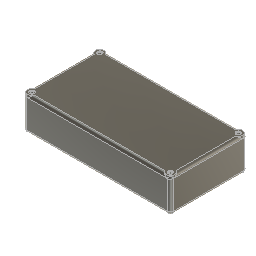
Meadow_Parametric_Enclosure (Autodesk Fusion 360 design; units mm, degrees)
Autodesk Fusion 360 part; units mm, degrees
sketch "Sketch1" plane through (0, 0, 0) normal (0, 0, 1) x (1, 0, 0) in component "Meadow_Enclosure_Bottom"
  line L0 (50, 25) -> (-50, 25)
  line L1 (-50, 25) -> (-50, -25)
  line L2 (-50, -25) -> (50, -25)
  line L3 (50, -25) -> (50, 25)
  line L4 (50, 25) -> (-50, -25) construction
  line L5 (-50, 25) -> (50, -25) construction
  line L6 (-52, -27) -> (52, -27)
  line L7 (52, -27) -> (52, 27)
  line L8 (52, 27) -> (-52, 27)
  line L9 (-52, 27) -> (-52, -27)
  dimension "d5" = 100
  dimension "d6" = 50
  dimension "d7" = 2
  constraint horizontal L0
  constraint perpendicular L0 L1
  constraint parallel L0 L2
  constraint parallel L1 L3
  constraint coincident L4 origin
  constraint coincident L5 origin
  measures "d5" distance of L1.end L2.end
  measures "d6" distance of L0.end L1.end
extrude "Extrude1" add sketch "Sketch1" along normal blind 2 contours L0 L1 L2 L3 makes body 1 in component "Meadow_Enclosure_Bottom"
extrude "Extrude2" add sketch "Sketch1" along normal blind 22 bodies 1 in component "Meadow_Enclosure_Bottom"
fillet "Fillet1" radius 2 8 edges at (-52, -27, 11) (-52, 27, 11) (52, -27, 11) (-52, 0, 0) (0, -27, 0) (0, 27, 0) (52, 0, 0) (52, 27, 11) on bodies 1 in component "Meadow_Enclosure_Bottom"
sketch "Sketch2" plane through (0, 0, 2) normal (0, 0, 1) x (-1, 0, 0) in component "Meadow_Enclosure_Bottom"
  line L0 (-50, 25) -> (-50, -25)
  line L1 (-50, -25) -> (50, -25)
  line L2 (50, -25) -> (50, 25)
  line L3 (50, 25) -> (-50, 25)
  line L4 (42.46, -25) -> (42.46, 25) construction
  line L5 (-50, 12.46) -> (50, 12.46) construction
  point P0 (42.46, 12.46)
  dimension "d148" = 7.54
  dimension "d149" = 12.54
  constraint coincident L1 L4.start
  constraint coincident L3 L4.end
  constraint perpendicular L3 L4
  constraint coincident L0 L5.start
  constraint coincident L2 L5.end
  constraint perpendicular L2 L5
  constraint coincident L4 P0
  constraint coincident L5 P0
  measures "d148" distance of L2.end L4
  measures "d149" distance of L2.end L5
sketch "Sketch6" plane through (0, 0, 22) normal (0, 0, 1) x (-1, 0, 0) in component "Meadow_Enclosure_Bottom"
  line L0 (-50, -25) -> (-50, 25)
  line L1 (-50, 25) -> (50, 25)
  line L2 (50, 25) -> (50, -25)
  line L3 (50, -25) -> (-50, -25)
  arc A0 (52, 25) -> (50, 27) centre (50, 25) ccw
  line L4 (50, 27) -> (-50, 27)
  arc A1 (-50, 27) -> (-52, 25) centre (-50, 25) ccw
  line L5 (-52, 25) -> (-52, -25)
  arc A2 (-52, -25) -> (-50, -27) centre (-50, -25) ccw
  line L6 (-50, -27) -> (50, -27)
  arc A3 (50, -27) -> (52, -25) centre (50, -25) ccw
  line L7 (52, -25) -> (52, 25)
  line L8 (-50, -25) -> (50, -25)
  line L9 (50, -25) -> (50, 25)
  circle A4 centre (49, -24) radius 3
  line L10 (-52, -27) -> (52, -27)
  line L11 (52, -27) -> (52, 27)
  circle A5 centre (49, 24) radius 3
  circle A6 centre (-49, 24) radius 3
  circle A7 centre (-49, -24) radius 3
  line L12 (52, 27) -> (-52, 27)
  line L13 (-52, 27) -> (-52, -27)
  constraint tangent A4 L10
  constraint tangent A4 L11
  constraint tangent L11 A5
  constraint tangent A5 L12
  constraint tangent A6 L13
  constraint tangent A6 L12
  constraint tangent L10 A7
  constraint tangent A7 L13
extrude "Extrude5" add sketch "Sketch6" against normal blind 4 contours L0 L3 L8 A7 | L0 L3 L8 A7 | L0 L1 A6 | L0 L1 A6 | L2 L3 L8 L9 A4 | L2 L3 L8 L9 A4 | L1 L2 L9 A5 | L1 L2 L9 A5 bodies 1 in component "Meadow_Enclosure_Bottom"
fillet "Fillet2" radius 1.5 16 edges at (46.1716, 25, 20) (50, 23.0858, 18) (48.0858, 25, 18) (50, 21.1716, 20) (50, -23.0858, 18) (48.0858, -25, 18) (46.1716, -25, 20) (50, -21.1716, 20) (-46.1716, -25, 20) (-50, -21.1716, 20) (-50, -23.0858, 18) (-48.0858, -25, 18) (-50, 23.0858, 18) (-48.0858, 25, 18) (-46.1716, 25, 20) (-50, 21.1716, 20) on bodies 1 in component "Meadow_Enclosure_Bottom"
hole "Hole2" at (-49, 24, 22) at (49, 24, 22) at (-49, -24, 22) at (49, -24, 22) direction (0, 0, -1) diameter 1.9 depth 3.75 tip angle 180 counterbore diameter 3.4 counterbore depth 3 bodies 1 in component "Meadow_Enclosure_Bottom"
sketch "PCB" plane through (0, 0, 0) normal (0, 0, 1) x (1, 0, 0) in component "Meadow_F7_Micro"
  line L0 (36.83, 11.43) -> (-36.83, 11.43)
  line L1 (-36.83, 11.43) -> (-36.83, -11.43)
  line L2 (-36.83, -11.43) -> (36.83, -11.43)
  line L3 (36.83, -11.43) -> (36.83, 11.43)
  line L4 (36.83, 11.43) -> (-36.83, -11.43) construction
  line L5 (-36.83, 11.43) -> (36.83, -11.43) construction
  circle A0 centre (-34.29, 8.89) radius 1.27
  circle A1 centre (-34.29, -8.89) radius 1.27
  line L6 (-36.83, 0) -> (36.83, 0) construction
  circle A2 centre (34.29, 8.89) radius 1.27
  circle A3 centre (34.29, -8.89) radius 1.27
  line L7 (0, 11.43) -> (0, -11.43) construction
  circle A4 centre (-13.97, 10.16) radius 0.51
  circle A5 centre (-11.43, 10.16) radius 0.51
  circle A6 centre (-8.89, 10.16) radius 0.51
  circle A7 centre (-6.35, 10.16) radius 0.51
  circle A8 centre (-3.81, 10.16) radius 0.51
  circle A9 centre (-1.27, 10.16) radius 0.51
  circle A10 centre (1.27, 10.16) radius 0.51
  circle A11 centre (3.81, 10.16) radius 0.51
  circle A12 centre (6.35, 10.16) radius 0.51
  circle A13 centre (8.89, 10.16) radius 0.51
  circle A14 centre (11.43, 10.16) radius 0.51
  circle A15 centre (13.97, 10.16) radius 0.51
  circle A16 centre (16.51, 10.16) radius 0.51
  circle A17 centre (19.05, 10.16) radius 0.51
  circle A18 centre (-24.13, -10.16) radius 0.51
  circle A19 centre (-21.59, -10.16) radius 0.51
  circle A20 centre (-19.05, -10.16) radius 0.51
  circle A21 centre (-16.51, -10.16) radius 0.51
  circle A22 centre (-13.97, -10.16) radius 0.51
  circle A23 centre (-11.43, -10.16) radius 0.51
  circle A24 centre (-8.89, -10.16) radius 0.51
  circle A25 centre (-6.35, -10.16) radius 0.51
  circle A26 centre (-3.81, -10.16) radius 0.51
  circle A27 centre (-1.27, -10.16) radius 0.51
  circle A28 centre (1.27, -10.16) radius 0.51
  circle A29 centre (3.81, -10.16) radius 0.51
  circle A30 centre (6.35, -10.16) radius 0.51
  circle A31 centre (8.89, -10.16) radius 0.51
  circle A32 centre (11.43, -10.16) radius 0.51
  circle A33 centre (13.97, -10.16) radius 0.51
  circle A34 centre (16.51, -10.16) radius 0.51
  circle A35 centre (19.05, -10.16) radius 0.51
  dimension "d1" = 73.66
  dimension "d2" = 22.86
  dimension "d3" = 2.54
  dimension "d4" = 2.54
  dimension "d5_1" = 2.54
  dimension "d7_1" = 2.54
  dimension "d8" = 1.02
  dimension "d9_1" = 20.32
  dimension "d10_1" = 1.27
  dimension "d13_1" = 2.54
  dimension "d14_1" = 0
  dimension "d15_1" = 1.02
  dimension "d16_1" = 10.16
  dimension "d17_1" = 1.27
  dimension "d20_1" = 2.54
  dimension "d21_1" = 0
  constraint horizontal L0
  constraint perpendicular L0 L1
  constraint parallel L0 L2
  constraint parallel L1 L3
  constraint coincident L4 origin
  constraint coincident L5 origin
  constraint midpoint L1 L6.start
  constraint midpoint L3 L6.end
  constraint symmetric A0.centre A1.centre L6
  constraint equal A0 A2
  constraint equal A0 A3
  constraint midpoint L0 L7.start
  constraint midpoint L2 L7.end
  constraint symmetric A0.centre A2.centre L7
  constraint symmetric A1.centre A3.centre L7
  measures "d1" distance of L1.end L2.end
  measures "d2" distance of L0.end L1.end
  measures "d3" diameter of A0
  measures "d4" distance of L0 A0.centre
  measures "d5_1" distance of L1 A0.centre
  measures "d7_1" diameter of A1
  measures "d8" diameter of A4
  measures "d9_1" horizontal distance of A0.centre A4.centre
  measures "d10_1" distance of L0 A4.centre
  measures "d15_1" diameter of A18
  measures "d16_1" horizontal distance of A1.centre A18.centre
  measures "d17_1" distance of L2 A18.centre
extrude "Extrude1'" add sketch "PCB" against normal blind 1.6 separate body makes body 2 in component "Meadow_F7_Micro"
fillet "Fillet1'" radius 2.54 4 edges at (-36.83, 11.43, -0.8) (-36.83, -11.43, -0.8) (36.83, -11.43, -0.8) (36.83, 11.43, -0.8) on bodies 2 in component "Meadow_F7_Micro"
sketch "Sketch4" plane through (0, 0, 0) normal (0, 0, 1) x (1, 0, 0) in component "Meadow_F7_Micro"
  line L0 (-36.83, 0) -> (36.83, 0) construction
  line L1 (-25.33, 10.93) -> (-18.08, 10.93)
  line L2 (-18.08, 10.93) -> (-18.08, 4.93)
  line L3 (-18.08, 4.93) -> (-25.33, 4.93)
  line L4 (-25.33, 4.93) -> (-25.33, 10.93)
  line L5 (-36.83, 11.43) -> (-36.83, -11.43)
  line L6 (36.83, 11.43) -> (-36.83, 11.43)
  line L7 (9.03, 5) -> (-0.97, 5)
  line L8 (-0.97, 5) -> (-0.97, -5)
  line L9 (-0.97, -5) -> (9.03, -5)
  line L10 (9.03, -5) -> (9.03, 5)
  line L11 (9.03, 5) -> (-0.97, -5) construction
  line L12 (-0.97, 5) -> (9.03, -5) construction
  line L13 (36.83, -11.43) -> (36.83, 11.43)
  line L14 (21.03, 4) -> (15.03, 4)
  line L15 (15.03, 4) -> (15.03, -4)
  line L16 (15.03, -4) -> (21.03, -4)
  line L17 (21.03, -4) -> (21.03, 4)
  line L18 (21.03, 4) -> (15.03, -4) construction
  line L19 (15.03, 4) -> (21.03, -4) construction
  line L20 (29.83, 3.5) -> (22.83, 3.5)
  line L21 (22.83, 3.5) -> (22.83, -3.5)
  line L22 (22.83, -3.5) -> (29.83, -3.5)
  line L23 (29.83, -3.5) -> (29.83, 3.5)
  line L24 (29.83, 3.5) -> (22.83, -3.5) construction
  line L25 (22.83, 3.5) -> (29.83, -3.5) construction
  line L26 (-7.47, -4) -> (-15.47, -4)
  line L27 (-15.47, -4) -> (-15.47, 4)
  line L28 (-15.47, 4) -> (-7.47, 4)
  line L29 (-7.47, 4) -> (-7.47, -4)
  line L30 (-7.47, -4) -> (-15.47, 4) construction
  line L31 (-15.47, -4) -> (-7.47, 4) construction
  line L32 (-22.17, -7.73) -> (-25.67, -7.73)
  line L33 (-25.67, -7.73) -> (-25.67, -1.23)
  line L34 (-25.67, -1.23) -> (-22.17, -1.23)
  line L35 (-22.17, -1.23) -> (-22.17, -7.73)
  line L36 (-22.17, -7.73) -> (-25.67, -1.23) construction
  line L37 (-25.67, -7.73) -> (-22.17, -1.23) construction
  line L38 (-36.83, -11.43) -> (36.83, -11.43)
  line L39 (-32.08, -4) -> (-37.83, -4)
  line L40 (-37.83, -4) -> (-37.83, 4)
  line L41 (-37.83, 4) -> (-32.08, 4)
  line L42 (-32.08, 4) -> (-32.08, -4)
  line L43 (-32.08, -4) -> (-37.83, 4) construction
  line L44 (-37.83, -4) -> (-32.08, 4) construction
  line L45 (34.63, 5.93) -> (36.23, 5.93)
  line L46 (36.23, 5.93) -> (36.23, 2.73)
  line L47 (36.23, 2.73) -> (34.63, 2.73)
  line L48 (34.63, 2.73) -> (34.63, 5.93)
  line L49 (28.23, -7.83) -> (30.83, -7.83)
  line L50 (30.83, -7.83) -> (30.83, -10.43)
  line L51 (30.83, -10.43) -> (28.23, -10.43)
  line L52 (28.23, -10.43) -> (28.23, -7.83)
  line L53 (21.18, 8.13) -> (25.33, 8.13)
  line L54 (25.33, 8.13) -> (25.33, 10.93)
  line L55 (25.33, 10.93) -> (21.18, 10.93)
  line L56 (21.18, 10.93) -> (21.18, 8.13)
  line L57 (21.18, -8.13) -> (25.33, -8.13)
  line L58 (25.33, -8.13) -> (25.33, -10.93)
  line L59 (25.33, -10.93) -> (21.18, -10.93)
  line L60 (21.18, -10.93) -> (21.18, -8.13)
  circle A0 centre (29.53, -9.13) radius 1
  point P0 (4.03, 0)
  point P1 (18.03, 0)
  point P2 (26.33, 0)
  point P3 (-11.47, 0)
  point P4 (-23.92, -4.48)
  point P5 (-34.955, 0)
  dimension "d25" = 7.25
  dimension "d26" = 6
  dimension "d27" = 11.5
  dimension "d28" = 0.5
  dimension "d29" = 10
  dimension "d30" = 10
  dimension "d31" = 27.8
  dimension "d32" = 6
  dimension "d33" = 8
  dimension "d34" = 6
  dimension "d35" = 7
  dimension "d36" = 7
  dimension "d37" = 1.8
  dimension "d38" = 8
  dimension "d39" = 8
  dimension "d40" = 6.5
  dimension "d41" = 3.5
  dimension "d42" = 6.5
  dimension "d43" = 3.7
  dimension "d44" = 6.7
  dimension "d45" = 5.75
  dimension "d46" = 8
  dimension "d47" = 4.75
  dimension "d48" = 1.6
  dimension "d49" = 3.2
  dimension "d50" = 5.5
  dimension "d51" = 0.6
  dimension "d52" = 2.6
  dimension "d53" = 2.6
  dimension "d54" = 1
  dimension "d55" = 6
  dimension "d56" = 4.15
  dimension "d57" = 2.8
  dimension "d58" = 11.5
  dimension "d59" = 0.5
  dimension "d60" = 4.15
  dimension "d61" = 2.8
  dimension "d62" = 11.5
  dimension "d63" = 0.5
  dimension "d64" = 2
  constraint horizontal L1
  constraint vertical L2
  constraint horizontal L3
  constraint vertical L4
  constraint horizontal L7
  constraint perpendicular L7 L8
  constraint parallel L7 L9
  constraint parallel L8 L10
  constraint coincident L11 P0
  constraint coincident L12 P0
  constraint coincident L0 P0
  constraint horizontal L14
  constraint perpendicular L14 L15
  constraint parallel L14 L16
  constraint parallel L15 L17
  constraint coincident L18 P1
  constraint coincident L19 P1
  constraint coincident L0 P1
  constraint horizontal L20
  constraint perpendicular L20 L21
  constraint parallel L20 L22
  constraint parallel L21 L23
  constraint coincident L24 P2
  constraint coincident L25 P2
  constraint coincident L0 P2
  constraint horizontal L26
  constraint perpendicular L26 L27
  constraint parallel L26 L28
  constraint parallel L27 L29
  constraint coincident L30 P3
  constraint coincident L31 P3
  constraint coincident L0 P3
  constraint horizontal L32
  constraint perpendicular L32 L33
  constraint parallel L32 L34
  constraint parallel L33 L35
  constraint coincident L36 P4
  constraint coincident L37 P4
  constraint horizontal L39
  constraint perpendicular L39 L40
  constraint parallel L39 L41
  constraint parallel L40 L42
  constraint coincident L43 P5
  constraint coincident L44 P5
  constraint horizontal L45
  constraint vertical L46
  constraint horizontal L47
  constraint vertical L48
  constraint horizontal L49
  constraint vertical L50
  constraint horizontal L51
  constraint vertical L52
  constraint horizontal L53
  constraint vertical L54
  constraint horizontal L55
  constraint vertical L56
  constraint horizontal L57
  constraint vertical L58
  constraint horizontal L59
  constraint vertical L60
  measures "d25" distance of L1.start L1.end
  measures "d26" distance of L1.start L3.end
  measures "d27" distance of L4 L5
  measures "d28" distance of L1 L6
  measures "d29" distance of L8.end L9.end
  measures "d30" distance of L7.end L8.end
  measures "d31" distance of L10 L13
  measures "d32" distance of L15.end L16.end
  measures "d33" distance of L14.end L15.end
  measures "d34" distance of L10 L15
  measures "d35" distance of L21.end L22.end
  measures "d36" distance of L20.end L21.end
  measures "d37" distance of L17 L21
  measures "d38" distance of L27.end L28.end
  measures "d39" distance of L26.end L27.end
  measures "d40" distance of L8 L29
  measures "d41" distance of L33.end L34.end
  measures "d42" distance of L32.end L33.end
  measures "d43" distance of L32 L38
  measures "d44" distance of L27 L35
  measures "d45" distance of L40.end L41.end
  measures "d46" distance of L39.end L40.end
  measures "d47" distance of L5 L42
  measures "d48" distance of L45.start L45.end
  measures "d49" distance of L45.start L47.end
  measures "d50" distance of L6 L45
  measures "d51" distance of L13 L46
  measures "d52" distance of L49.start L49.end
  measures "d53" distance of L49.start L51.end
  measures "d54" distance of L38 L51
  measures "d55" distance of L13 L50
  measures "d56" distance of L53.start L53.end
  measures "d57" distance of L53.start L55.end
  measures "d58" distance of L13 L54
  measures "d59" distance of L6 L55
  measures "d60" distance of L57.start L57.end
  measures "d61" distance of L57.start L59.end
  measures "d62" distance of L13 L58
  measures "d63" distance of L38 L59
  measures "d64" diameter of A0
extrude "Extrude2'" add sketch "Sketch4" along normal blind 1 separate body contours L26 L27 L28 L29 makes body 3 in component "Meadow_F7_Micro"
extrude "Extrude3" add sketch "Sketch4" along normal blind 0.6 separate body contours L7 L8 L9 L10 makes body 4 in component "Meadow_F7_Micro"
extrude "Extrude4" add sketch "Sketch4" along normal blind 1 separate body contours L14 L15 L16 L17 makes body 5 in component "Meadow_F7_Micro"
extrude "Extrude5'" add sketch "Sketch4" along normal blind 0.9 separate body contours L20 L21 L22 L23 makes body 6 in component "Meadow_F7_Micro"
extrude "Extrude6" add sketch "Sketch4" along normal blind 1.2 separate body contours L45 L46 L47 L48 makes body 7 in component "Meadow_F7_Micro"
extrude "Extrude7" add sketch "Sketch4" along normal blind 5.4 separate body contours L1 L2 L3 L4 makes body 8 in component "Meadow_F7_Micro"
extrude "Extrude8" add sketch "Sketch4" along normal blind 2.5 separate body contours L5 L39 L41 L42 | L5 L39 L40 L41 makes body 9 in component "Meadow_F7_Micro"
extrude "Extrude9" add sketch "Sketch4" along normal blind 1.5 separate body contours L32 L33 L34 L35 makes body 10 in component "Meadow_F7_Micro"
extrude "Extrude10" add sketch "Sketch4" along normal blind 0.4 separate body contours L49 L50 L51 L52 makes body 11 in component "Meadow_F7_Micro"
extrude "Extrude11" add sketch "Sketch4" along normal blind 1.5 contours A0 bodies 9 10 8 2 11 in component "Meadow_F7_Micro"
extrude "Extrude12" add sketch "Sketch4" along normal blind 1.5 separate body contours L53 L54 L55 L56 makes body 12 in component "Meadow_F7_Micro"
extrude "Extrude13" add sketch "Sketch4" along normal blind 1.5 separate body contours L57 L58 L59 L60 makes body 13 in component "Meadow_F7_Micro"
sketch "Sketch1 (2)" plane through (0, 0, -1.6) normal (0, 0, -1) x (1, 0, 0) in component "Meadow_F7_Micro v7"
  arc A0 (34.29, -11.43) -> (36.83, -8.89) centre (34.29, -8.89) ccw
  line L0 (36.83, -8.89) -> (36.83, 8.89)
  arc A1 (36.83, 8.89) -> (34.29, 11.43) centre (34.29, 8.89) ccw
  line L1 (34.29, 11.43) -> (-34.29, 11.43)
  arc A2 (-34.29, 11.43) -> (-36.83, 8.89) centre (-34.29, 8.89) ccw
  line L2 (-36.83, 8.89) -> (-36.83, -8.89)
  arc A3 (-36.83, -8.89) -> (-34.29, -11.43) centre (-34.29, -8.89) ccw
  line L3 (-34.29, -11.43) -> (34.29, -11.43)
  circle A4 centre (-3.81, 10.16) radius 0.51
  circle A5 centre (11.43, -10.16) radius 0.51
  circle A6 centre (-19.05, 10.16) radius 0.51
  circle A7 centre (19.05, -10.16) radius 0.51
  circle A8 centre (34.29, 8.89) radius 1.27
  circle A9 centre (11.43, 10.16) radius 0.51
  circle A10 centre (-24.13, 10.16) radius 0.51
  circle A11 centre (-8.89, 10.16) radius 0.51
  circle A12 centre (-21.59, 10.16) radius 0.51
  circle A13 centre (6.35, 10.16) radius 0.51
  circle A14 centre (-34.29, -8.89) radius 1.27
  circle A15 centre (-34.29, 8.89) radius 1.27
  circle A16 centre (16.51, -10.16) radius 0.51
  circle A17 centre (-11.43, -10.16) radius 0.51
  circle A18 centre (-11.43, 10.16) radius 0.51
  circle A19 centre (-13.97, -10.16) radius 0.51
  circle A20 centre (13.97, -10.16) radius 0.51
  circle A21 centre (-8.89, -10.16) radius 0.51
  circle A22 centre (16.51, 10.16) radius 0.51
  circle A23 centre (1.27, 10.16) radius 0.51
  circle A24 centre (-6.35, 10.16) radius 0.51
  circle A25 centre (13.97, 10.16) radius 0.51
  circle A26 centre (6.35, -10.16) radius 0.51
  circle A27 centre (8.89, 10.16) radius 0.51
  circle A28 centre (-13.97, 10.16) radius 0.51
  circle A29 centre (19.05, 10.16) radius 0.51
  circle A30 centre (-16.51, 10.16) radius 0.51
  circle A31 centre (-1.27, 10.16) radius 0.51
  circle A32 centre (8.89, -10.16) radius 0.51
  circle A33 centre (3.81, 10.16) radius 0.51
  circle A34 centre (34.29, -8.89) radius 1.27
  circle A35 centre (1.27, -10.16) radius 0.51
  circle A36 centre (-6.35, -10.16) radius 0.51
  circle A37 centre (-3.81, -10.16) radius 0.51
  circle A38 centre (3.81, -10.16) radius 0.51
  circle A39 centre (-1.27, -10.16) radius 0.51
  point P0 (34.29, 8.89)
sketch "Sketch1 (3)" plane through (0, 0, -1.6) normal (0, 0, -1) x (1, 0, 0) in component "Clearance"
  line L0 (-36.83, 11.43) -> (36.83, 11.43)
  line L1 (36.83, 11.43) -> (36.83, -11.43)
  line L2 (36.83, -11.43) -> (-36.83, -11.43)
  line L3 (-36.83, -11.43) -> (-36.83, 11.43)
  point P0 (-36.83, 11.43)
  point P1 (36.83, -11.43)
  constraint horizontal L0
  constraint vertical L1
  constraint horizontal L2
  constraint vertical L3
  constraint coincident P1 L1.end
  constraint coincident P0 L0.start
extrude "Extrude1''" add sketch "Sketch1 (3)" along normal blind 2 separate body makes body 14 in component "Clearance"
fillet "Fillet1''" radius 2.54 4 edges at (-36.83, -11.43, -2.6) (36.83, -11.43, -2.6) (36.83, 11.43, -2.6) (-36.83, 11.43, -2.6) on bodies 14 in component "Clearance"
sketch "Sketch2 (2)" plane through (-37.83, 0, 0) normal (-1, 0, 0) x (0, -1, 0) in component "Clearance"
  line L0 (-4, 0) -> (4, 0)
  line L1 (4, 0) -> (4, 2.5)
  line L2 (4, 2.5) -> (-4, 2.5)
  line L3 (-4, 2.5) -> (-4, 0)
  line L4 (0, 2.5) -> (0, 0) construction
  line L5 (-4, 1.25) -> (4, 1.25) construction
  line L6 (6, 4.75) -> (-6, 4.75)
  line L7 (-6, 4.75) -> (-6, -2.25)
  line L8 (-6, -2.25) -> (6, -2.25)
  line L9 (6, -2.25) -> (6, 4.75)
  line L10 (6, 4.75) -> (-6, -2.25) construction
  line L11 (-6, 4.75) -> (6, -2.25) construction
  point P0 (0, 1.25)
  dimension "d96" = 12
  dimension "d97" = 7
  constraint midpoint L2 L4.start
  constraint coincident L4.end origin
  constraint midpoint L3 L5.start
  constraint midpoint L1 L5.end
  constraint horizontal L6
  constraint perpendicular L6 L7
  constraint parallel L6 L8
  constraint parallel L7 L9
  constraint coincident L10 P0
  constraint coincident L11 P0
  constraint midpoint L4 P0
  measures "d96" distance of L7.end L8.end
  measures "d97" distance of L6.end L7.end
extrude "Extrude2''" add sketch "Sketch2 (2)" along normal blind 16 separate body contours L0 L1 L2 L3 | L6 L7 L8 L9 makes body 15 in component "Clearance"
sketch "Sketch3" plane through (0, 0, -3.6) normal (0, 0, -1) x (1, 0, 0) in component "Clearance"
  arc A0 (-36.83, -8.89) -> (-34.29, -11.43) centre (-34.29, -8.89) ccw
  line L0 (-34.29, -11.43) -> (34.29, -11.43)
  arc A1 (34.29, -11.43) -> (36.83, -8.89) centre (34.29, -8.89) ccw
  line L1 (36.83, -8.89) -> (36.83, 8.89)
  arc A2 (36.83, 8.89) -> (34.29, 11.43) centre (34.29, 8.89) ccw
  line L2 (34.29, 11.43) -> (-34.29, 11.43)
  arc A3 (-34.29, 11.43) -> (-36.83, 8.89) centre (-34.29, 8.89) ccw
  line L3 (-36.83, 8.89) -> (-36.83, -8.89)
  point P0 (-34.29, 8.89)
  point P1 (-34.29, -8.89)
  point P2 (34.29, 8.89)
  point P3 (34.29, -8.89)
sketch "Sketch4 (2)" plane through (0, 0, 0) normal (0, 0, 1) x (1, 0, 0) in component "Clearance"
  line L0 (36.83, -11.43) -> (-36.83, -11.43)
  line L1 (-36.83, -11.43) -> (-36.83, 11.43)
  line L2 (-36.83, 11.43) -> (36.83, 11.43)
  line L3 (36.83, 11.43) -> (36.83, -11.43)
  point P0 (-36.83, 11.43)
  point P1 (36.83, -11.43)
  constraint horizontal L0
  constraint vertical L1
  constraint horizontal L2
  constraint vertical L3
  constraint coincident P0 L1.end
  constraint coincident P1 L0.start
extrude "Extrude3'" add sketch "Sketch4 (2)" along normal blind 8.5 separate body makes body 16 in component "Clearance"
fillet "Fillet2'" radius 2.54 4 edges at (-36.83, -11.43, 4.25) (36.83, -11.43, 4.25) (-36.83, 11.43, 4.25) (36.83, 11.43, 4.25) on bodies 16 in component "Clearance"
sketch "Sketch1 (4)" plane through (0, 0, 22) normal (0, 0, 1) x (-1, 0, 0) in component "Meadow_Enclosure_Top"
  circle A0 centre (49, 24) radius 1.7
  circle A1 centre (49, -24) radius 1.7
  circle A2 centre (-49, -24) radius 1.7
  circle A3 centre (-49, 24) radius 1.7
  line L0 (44.5279, -25) -> (-44.5279, -25)
  arc A4 (-46.0186, -23.6667) -> (-44.5279, -25) centre (-44.5279, -23.5) ccw
  arc A5 (-46.0186, -23.6667) -> (-48.6667, -21.0186) centre (-49, -24) ccw
  arc A6 (-50, -19.5279) -> (-48.6667, -21.0186) centre (-48.5, -19.5279) ccw
  line L1 (-50, -19.5279) -> (-50, 19.5279)
  arc A7 (-48.6667, 21.0186) -> (-50, 19.5279) centre (-48.5, 19.5279) ccw
  arc A8 (-48.6667, 21.0186) -> (-46.0186, 23.6667) centre (-49, 24) ccw
  arc A9 (-44.5279, 25) -> (-46.0186, 23.6667) centre (-44.5279, 23.5) ccw
  line L2 (-44.5279, 25) -> (44.5279, 25)
  arc A10 (46.0186, 23.6667) -> (44.5279, 25) centre (44.5279, 23.5) ccw
  arc A11 (46.0186, 23.6667) -> (48.6667, 21.0186) centre (49, 24) ccw
  arc A12 (50, 19.5279) -> (48.6667, 21.0186) centre (48.5, 19.5279) ccw
  line L3 (50, 19.5279) -> (50, -19.5279)
  arc A13 (48.6667, -21.0186) -> (50, -19.5279) centre (48.5, -19.5279) ccw
  arc A14 (48.6667, -21.0186) -> (46.0186, -23.6667) centre (49, -24) ccw
  arc A15 (44.5279, -25) -> (46.0186, -23.6667) centre (44.5279, -23.5) ccw
  line L4 (-50, -27) -> (50, -27)
  arc A16 (50, -27) -> (52, -25) centre (50, -25) ccw
  line L5 (52, -25) -> (52, 25)
  arc A17 (52, 25) -> (50, 27) centre (50, 25) ccw
  line L6 (50, 27) -> (-50, 27)
  arc A18 (-50, 27) -> (-52, 25) centre (-50, 25) ccw
  line L7 (-52, 25) -> (-52, -25)
  arc A19 (-52, -25) -> (-50, -27) centre (-50, -25) ccw
  arc A20 (-45.7701, -23.6389) -> (-44.5279, -24.75) centre (-44.5279, -23.5) ccw
  line L8 (44.5279, -24.75) -> (-44.5279, -24.75)
  arc A21 (44.5279, -24.75) -> (45.7701, -23.6389) centre (44.5279, -23.5) ccw
  arc A22 (48.6389, -20.7701) -> (45.7701, -23.6389) centre (49, -24) ccw
  arc A23 (48.6389, -20.7701) -> (49.75, -19.5279) centre (48.5, -19.5279) ccw
  line L9 (49.75, 19.5279) -> (49.75, -19.5279)
  arc A24 (49.75, 19.5279) -> (48.6389, 20.7701) centre (48.5, 19.5279) ccw
  arc A25 (45.7701, 23.6389) -> (48.6389, 20.7701) centre (49, 24) ccw
  arc A26 (45.7701, 23.6389) -> (44.5279, 24.75) centre (44.5279, 23.5) ccw
  line L10 (-44.5279, 24.75) -> (44.5279, 24.75)
  arc A27 (-44.5279, 24.75) -> (-45.7701, 23.6389) centre (-44.5279, 23.5) ccw
  arc A28 (-48.6389, 20.7701) -> (-45.7701, 23.6389) centre (-49, 24) ccw
  arc A29 (-48.6389, 20.7701) -> (-49.75, 19.5279) centre (-48.5, 19.5279) ccw
  line L11 (-49.75, -19.5279) -> (-49.75, 19.5279)
  arc A30 (-49.75, -19.5279) -> (-48.6389, -20.7701) centre (-48.5, -19.5279) ccw
  arc A31 (-45.7701, -23.6389) -> (-48.6389, -20.7701) centre (-49, -24) ccw
  line L12 (43.901, -22.75) -> (-43.901, -22.75)
  arc A32 (-43.901, -22.75) -> (-47.75, -18.901) centre (-49, -24) ccw
  line L13 (-47.75, -18.901) -> (-47.75, 18.901)
  arc A33 (-47.75, 18.901) -> (-43.901, 22.75) centre (-49, 24) ccw
  line L14 (-43.901, 22.75) -> (43.901, 22.75)
  arc A34 (43.901, 22.75) -> (47.75, 18.901) centre (49, 24) ccw
  line L15 (47.75, 18.901) -> (47.75, -18.901)
  arc A35 (47.75, -18.901) -> (43.901, -22.75) centre (49, -24) ccw
  point P0 (49, -24)
  point P1 (49, 24)
  point P2 (-49, 24)
  point P3 (-49, -24)
  dimension "d198" = 0.25
  dimension "d199" = -2.25
extrude "Extrude1'''" add sketch "Sketch1 (4)" along normal blind 2 separate body contours A0 | A1 | A2 | A3 | L0 A4 A5 A6 L1 A7 A8 A9 L2 A10 A11 A12 L3 A13 A14 A15 | L4 A16 L5 A17 L6 A18 L7 A19 | A20 L8 A21 A22 A23 L9 A24 A25 A26 L10 A27 A28 A29 L11 A30 A31 | L12 A32 L13 A33 L14 A34 L15 A35 makes body 17 in component "Meadow_Enclosure_Top"
extrude "Extrude2'''" add sketch "Sketch1 (4)" against normal blind 2 contours A20 L8 A21 A22 A23 L9 A24 A25 A26 L10 A27 A28 A29 L11 A30 A31 bodies 17 in component "Meadow_Enclosure_Top"
sketch "Sketch2 (3)" plane through (0, 0, 24) normal (0, 0, 1) x (-1, 0, 0) in component "Meadow_Enclosure_Top"
  arc A0 (-52, -25) -> (-50, -27) centre (-50, -25) ccw
  line L0 (-50, -27) -> (50, -27)
  arc A1 (50, -27) -> (52, -25) centre (50, -25) ccw
  line L1 (52, -25) -> (52, 25)
  arc A2 (52, 25) -> (50, 27) centre (50, 25) ccw
  line L2 (50, 27) -> (-50, 27)
  arc A3 (-50, 27) -> (-52, 25) centre (-50, 25) ccw
  line L3 (-52, 25) -> (-52, -25)
  circle A4 centre (49, -24) radius 3
  circle A5 centre (49, 24) radius 3
  circle A6 centre (-49, -24) radius 3
  circle A7 centre (-49, 24) radius 3
  circle A8 centre (49, -24) radius 3
  point P0 (49, -24)
  point P1 (49, 24)
  point P2 (-49, 24)
  point P3 (-49, -24)
  constraint coincident P0 A4.centre
  constraint coincident P1 A5.centre
  constraint coincident P3 A6.centre
  constraint coincident P2 A7.centre
  constraint equal A4 A8
  constraint equal A4 A5
  constraint equal A4 A6
  constraint equal A4 A7
fillet "Fillet1'''" radius 2 8 edges at (52, 0, 24) (51.4142, 26.4142, 24) (0, 27, 24) (-51.4142, 26.4142, 24) (-52, 0, 24) (-51.4142, -26.4142, 24) (0, -27, 24) (51.4142, -26.4142, 24) on bodies 17 in component "Meadow_Enclosure_Top"
extrude "Extrude3''" add sketch "Sketch2 (3)" against normal up to surface (2 mm away) contours A6 | A7 | A4 A8 | A5 bodies 17 in component "Meadow_Enclosure_Top"
hole "Hole1" at (-49, 24, 24) at (-49, -24, 24) at (49, -24, 24) at (49, 24, 24) direction (0, 0, -1) diameter 1.9 depth 4.5 tip angle 180 counterbore diameter 3.4 counterbore depth 0.5 bodies 17 in component "Meadow_Enclosure_Top"
sketch "Sketch9" plane through (0, 0, 2) normal (0, 0, 1) x (-1, 0, 0) in component "Meadow_Enclosure_Bottom"
  circle A0 centre (42.46, 12.46) radius 3
  circle A1 centre (42.46, -5.32) radius 3
  circle A2 centre (-26.12, -5.32) radius 3
  circle A3 centre (-26.12, 12.46) radius 3
  point P0 (-26.12, -5.32)
  point P1 (-26.12, 12.46)
  point P2 (42.46, -5.32)
  point P3 (42.46, 12.46)
  dimension "d184" = 6
  constraint coincident P3 A0.centre
  constraint coincident P2 A1.centre
  constraint coincident P0 A2.centre
  constraint coincident P1 A3.centre
  constraint equal A0 A1
  constraint equal A0 A2
  constraint equal A0 A3
  measures "d184" diameter of A0
extrude "Extrude7'" add sketch "Sketch9" along normal up to surface (2 mm away) bodies 1 in component "Meadow_Enclosure_Bottom"
sketch "Sketch10" plane through (0, 0, 4) normal (0, 0, 1) x (-1, 0, 0) in component "Meadow_Enclosure_Bottom"
  circle A0 centre (-26.12, 12.46) radius 3
  point P0 (42.46, -5.32)
  point P1 (42.46, 12.46)
  point P2 (-26.12, -5.32)
  point P3 (-26.12, 12.46)
hole "Hole4" at (26.12, -12.46, 4) at (26.12, 5.32, 4) at (-42.46, 5.32, 4) at (-42.46, -12.46, 4) direction (0, 0, -1) diameter 1.9 depth 3.75 tip angle 180 counterbore diameter 3.4 counterbore depth 3 bodies 1 in component "Meadow_Enclosure_Bottom"
chamfer "Chamfer3" distance 0.2 distance2 3 4 edges at (24.535, -11.8453, 4) (-44.045, -11.8453, 4) (-44.045, 5.9347, 4) (24.535, 5.9347, 4) measured on face at (23.5661, -12.2686, 4) measured on face at (-45.0139, -12.2686, 4) measured on face at (-45.0139, 5.5114, 4) measured on face at (23.5661, 5.5114, 4) on bodies 1 in component "Meadow_Enclosure_Bottom"
sketch "Sketch11" plane through (-52, 0, 0) normal (-1, 0, 0) x (0, -1, 0) in component "Meadow_Enclosure_Bottom"
  line L0 (25, 2) -> (25, 22)
  line L1 (25, 22) -> (-25, 22)
  line L2 (-25, 22) -> (-25, 2)
  line L3 (-25, 2) -> (25, 2)
  line L4 (9.57, 3.35) -> (9.57, 10.35)
  line L5 (9.57, 10.35) -> (-2.43, 10.35)
  line L6 (-2.43, 10.35) -> (-2.43, 3.35)
  line L7 (-2.43, 3.35) -> (9.57, 3.35)
extrude "Extrude8'" cut sketch "Sketch11" against normal up to surface (2 mm away) contours L4 L5 L6 L7 bodies 1 in component "Meadow_Enclosure_Bottom"
component "Meadow_Enclosure_Bottom" placed x (1, 0, 0) y (0, 1, 0) z (0, 0, 1) at (0, 0, 0)
component "Meadow_F7_Micro v7" placed x (1, 0, 0) y (0, 1, 0) z (0, 0, 1) at (0, 0, 0)
component "Meadow_Enclosure_Top" placed x (1, 0, 0) y (0, 1, 0) z (0, 0, 1) at (0, 0, 0)
component "Meadow_F7_Micro" placed x (1, 0, 0) y (0, 1, 0) z (0, 0, 1) at (-8.17, -3.57, 5.6) in component "Meadow_F7_Micro v7"
component "Clearance" placed x (1, 0, 0) y (0, 1, 0) z (0, 0, 1) at (-8.17, -3.57, 5.6) in component "Meadow_F7_Micro v7"
equation "InternalWidth = 100 mm"
equation "InternalDepth = 50 mm"
equation "InternalHeight = 20 mm"
equation "WallThickness = 2 mm"
equation "d5 = InternalWidth"
equation "d6 = InternalDepth"
equation "d7 = WallThickness"
equation "ExternalChamfer = WallThickness" comment "Must be <= Wall Thickness"
equation "d9 = WallThickness"
equation "d11 = InternalHeight + WallThickness"
equation "d22 = ExternalChamfer"
equation "Meadow_X = 5 mm" comment "Must be > ~0.5mm"
equation "Meadow_Y = 10 mm" comment "Must be > ~0.5mm"
equation "d148 = Meadow_X + 2.54 mm"
equation "d149 = Meadow_Y + 2.54 mm"
equation "d7_1 = d3"
equation "d17_1 = d10_1"
equation "d62 = d58"
equation "d63 = d59"
equation "d199 = -( ExternalChamfer + 0.25 mm )"
equation "d200 = WallThickness"
equation "d204 = ExternalChamfer"
equation "d210 = WallThickness - 1.5 mm"
named bodies: "PCB", "RAM", "ESP32", "Antenny", "Flash", "F7", "Battery_Conn", "USB_Conn", "Power_Buck", "Reset_Btn", "Boot_Btn"
